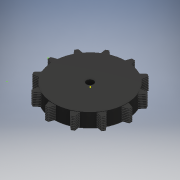
# Autodesk Inventor part: spiked-wheel
Saved by Autodesk Inventor 2018 (Build 220112000, 112)
## iProperties
Created: 2018-01-20
Part Number: spiked-wheel
Material: Rubber
Document SubType Name: Modeling
Designer: Ahmed
Density: 0.93 g/cm^3
Appearance: Rubber - Black
Author: Ahmed
Autodesk Inventor part; units mm, degrees
ref_plane "YZ Plane" through (0, 0, 0) normal (1, 0, 0) x (0, 1, 0)
ref_plane "XZ Plane" through (0, 0, 0) normal (0, 1, 0) x (-1, 0, 0)
ref_plane "XY Plane" through (0, 0, 0) normal (0, 0, 1) x (1, 0, 0)
sketch "Sketch1" plane through (0, 0, 0) normal (0, 0, 1) x (1, 0, 0)
  circle A0 centre (-64.4824, 58.0834) radius 500
  point P0 (0, 0)
  dimension "d0" = 1000
  constraints: 1 centre point
  measures "d0" diameter of A0
sketch "Sketch2" plane through (0, 0, 0) normal (0, 0, 1) x (1, 0, 0)
  point P0 (0, 0)
extrude "Extrusion1" add sketch "Sketch1" along normal blind 200
sketch "Sketch3" plane through (-64.4824, 58.0834, 200) normal (0, 0, 1) x (1, 0, 0)
  circle A0 centre (0, 0) radius 500 projected
  line L0 (0, 500) -> (65.5119, 500)
  line L1 (0, 500) -> (-31.0013, 499.038)
  line L2 (-31.0013, 499.038) -> (-2.6124, 577.0358)
  line L3 (-31.0013, 499.038) -> (52.0022, 499.038) construction
  line L4 (65.5119, 500) -> (37.4731, 577.0358)
  line L5 (65.5119, 500) -> (147.4917, 500) construction
  line L6 (-2.6124, 577.0358) -> (37.4731, 577.0358)
  point P0 (64.4824, -58.0834)
  constraints: 14 end point, 4 horizontal, 2 equal length, 2 point on circle, 1 tangent
extrude "Extrusion2" add sketch "Sketch3" along normal mid plane 10 contours A0 L2 L6 L4 L0
sketch "Sketch4" plane through (-27.0093, 635.1192, 205) normal (0.9396926, 0.3420201, 0) x (0, 0, -1)
  point P0 (205, -606.0545)
sketch "Sketch5" plane through (0, 0, 200) normal (0, 0, 1) x (1, 0, 0)
  point P0 (0, 0)
sketch "Sketch6" plane through (-27.0093, 635.1192, 205) normal (0.9396926, 0.3420201, 0) x (0, 0, -1)
  line L0 (10, -81.9798) -> (0, -81.9798) projected
  line L1 (0, 0) -> (0, 13.7101) projected
  line L2 (5, -81.9798) -> (0, -81.9798)
  line L3 (0, -81.9798) -> (0, 13.7101)
  line L4 (0, 13.7101) -> (5, 13.7101)
  line L5 (5, 13.7101) -> (5, -81.9798)
  point P0 (205, -606.0545)
  constraints: 8 end point, 2 parallel, 1 horizontal, 1 midpoint, 1 perpendicular
extrude "Extrusion3" cut sketch "Sketch6" against normal blind 20
pattern_linear "Rectangular Pattern1" count 10 spacing 20 along (0, 0, -1) of "Extrusion2"
sketch "Sketch7" plane through (1.0295, 558.0834, 200) normal (0.9396926, 0.3420201, 0) x (0, 0, -1)
  point P0 (200, -524.0747)
sketch "Sketch8" plane through (0, 0, 200) normal (0, 0, 1) x (1, 0, 0)
  point P0 (0, 0)
sketch "Sketch9" plane through (1.0295, 558.0834, 200) normal (0.9396926, 0.3420201, 0) x (0, 0, -1)
  point P0 (200, -524.0747)
sketch "Sketch10" plane through (1.0295, 558.0834, 200) normal (0.9396926, 0.3420201, 0) x (0, 0, -1)
  point P0 (200, -524.0747)
sketch "Sketch11" plane through (0, 0, 200) normal (0, 0, 1) x (1, 0, 0)
  point P0 (0, 0)
pattern_circular "Circular Pattern1" count 12 over 360 about axis through (-64.4824, 58.0834, 0) along (0, 0, 1) of "Extrusion2", "Rectangular Pattern1", "Extrusion1"
sketch "Sketch12" plane through (-64.4824, 558.0834, 165) normal (0, -1, 0) x (1, 0, 0)
  line L0 (-577.0358, 30) -> (-577.0358, 40) projected
  line L1 (500, 40) -> (577.0358, 40) projected
  line L2 (-577.0358, 30) -> (577.0358, 30)
  line L3 (577.0358, 30) -> (577.0358, 40)
  line L4 (577.0358, 40) -> (-577.0358, 40)
  line L5 (-577.0358, 40) -> (-577.0358, 30)
  point P0 (64.4824, -165)
  constraints: 8 end point, 2 parallel, 1 horizontal, 1 perpendicular
extrude "Extrusion4" cut sketch "Sketch12" along normal mid plane 1000
sketch "Sketch13" plane through (-64.4824, 58.0834, 195) normal (0, 0, 1) x (-1, 0, 0)
  circle A0 centre (0, 0) radius 50
  point P0 (-64.4824, 58.0834)
  dimension "d30" = 100
  constraints: 1 centre point
  measures "d30" diameter of A0
extrude "Extrusion5" cut sketch "Sketch13" against normal blind 200
sketch "Sketch14" plane through (0, 0, 200) normal (0, 0, 1) x (1, 0, 0)
  point P0 (0, 0)
sketch "Sketch15" plane through (-641.5182, 55.471, 195) normal (-1, 0, 0) x (0, 0, 1)
  line L0 (0, 0) -> (10, 0)
  line L1 (10, -563.86) -> (0, -563.86)
  point P0 (-195, -55.471)
  constraints: 4 end point, 1 horizontal, 1 parallel
sketch "Sketch16" plane through (-641.5182, 55.471, 195) normal (-0.3420201, -0.9396926, 0) x (0.9396926, -0.3420201, 0)
  line L0 (1110.0657, 0) -> (1110.0657, 10) projected
  line L1 (1110.0657, 0) -> (-9.9849, 0)
  line L2 (-9.9849, 0) -> (-9.9849, 15.7317)
  line L3 (-9.9849, 15.7317) -> (1110.0657, 15.7317)
  line L4 (1110.0657, 15.7317) -> (1110.0657, 0)
  point P0 (621.8021, -195)
  constraints: 8 end point, 2 parallel, 1 horizontal, 1 perpendicular
extrude "Extrusion6" cut sketch "Sketch16" along normal mid plane 2000
sketch "Sketch17" plane through (-64.4824, 58.0834, 195) normal (0, 0, 1) x (1, 0, 0)
  point P0 (64.4824, -58.0834)
body "Solid1"
